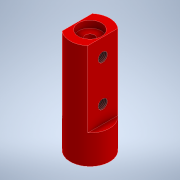
# Autodesk Inventor part: Drum
Saved by Autodesk Inventor 2021 (Build 250183000, 183)
## iProperties
Created: 2022-05-14
Part Number: Drum
Material: Aluminum 6061
Document SubType Name: Modeling
Designer: ermoz
Density: 2.7 g/cm^3
Appearance: Aluminum - Flat
Mass: 135.109 g
Surface Area: 148.591 cm^2
Volume: 50.0405 cm^3
Author: ermoz
Autodesk Inventor part; units mm, degrees
ref_plane "YZ Plane" through (0, 0, 0) normal (1, 0, 0) x (0, 1, 0)
ref_plane "XZ Plane" through (0, 0, 0) normal (0, 1, 0) x (-1, 0, 0)
ref_plane "XY Plane" through (0, 0, 0) normal (0, 0, 1) x (1, 0, 0)
sketch "Sketch1" plane through (0, 0, 0) normal (0, 1, 0) x (-1, 0, 0)
  circle A0 centre (0, 0) radius 4
  circle A1 centre (0, 0) radius 17
  dimension "d0" = 8
  dimension "d1" = 34
  constraints: 2 centre point, 2 coincident
  measures "d0" diameter of A0
  measures "d1" diameter of A1
extrude "Extrusion1" add sketch "Sketch1" along normal blind 90
sketch "Sketch3" plane through (0, 90, 0) normal (0, 1, 0) x (1, 0, 0)
  line L0 (11, 24.9102) -> (-11, 24.9102)
  line L1 (-11, 24.9102) -> (-11, -24.9102)
  line L2 (-11, -24.9102) -> (11, -24.9102)
  line L3 (11, -24.9102) -> (11, 24.9102)
  line L4 (11, 24.9102) -> (-11, -24.9102) construction
  line L5 (-11, 24.9102) -> (11, -24.9102) construction
  circle A0 centre (0, 0) radius 17
  circle A1 centre (0, 0) radius 17 projected
  point P0 (11, 12.9615)
  point P1 (11, -12.9615)
  point P2 (-11, -12.9615)
  point P3 (-11, 12.9615)
  dimension "d7" = 22
  constraints: 12 end point, 2 midpoint, 2 parallel, 1 centre point, 1 coincident, 1 concentric, 1 horizontal, 1 perpendicular
  measures "d7" distance of L1.end L2.end
extrude "Extrusion3" cut sketch "Sketch3" against normal blind 65 contours A0 L3 | L1 A0
sketch "Sketch4" plane through (-11, 90, -12.9615) normal (-1, 0, 0) x (0, 0, 1)
  circle A0 centre (12.9615, -50) radius 4
  circle A1 centre (12.9615, -15) radius 4
  line L0 (0, 0) -> (25.923, 0) projected
  line L1 (29.9615, -90) -> (-4.0385, -90) projected
  line L2 (0, -65) -> (25.923, -65) projected
  line L3 (25.923, 0) -> (25.923, -65) projected
  line L4 (0, 0) -> (25.923, 0) projected
  line L5 (0, -65) -> (0, 0) projected
  line L6 (0, -65) -> (25.923, -65) projected
  line L7 (25.923, 0) -> (25.923, -65) projected
  line L8 (12.9615, -65) -> (12.9615, -59.6994)
  point P0 (0.995, 0)
  point P1 (15.5881, 0)
  dimension "d12" = 15
  dimension "d15" = 8
  dimension "d17" = 15
  constraints: 2 centre point, 2 end point, 1 equal radius, 1 midpoint, 1 point on line, 1 vertical, 1 vertical alignment
  measures "d12" distance from line of L0 A1.centre
  measures "d15" diameter of A0
  measures "d17" distance from line of L2 A0.centre
extrude "Extrusion4" cut sketch "Sketch4" against normal through all contours A0 | A1
sketch "Sketch5" plane through (0, 0, 0) normal (0, -1, 0) x (1, 0, 0)
  circle A0 centre (0, 0) radius 14.5
  dimension "d18" = 29
  constraints: 1 centre point, 1 coincident
  measures "d18" diameter of A0
extrude "Extrusion5" cut sketch "Sketch5" against normal blind 18
thread "Thread1" size "M8x1.25" class "6H" standard "ANSI Metric M Profile" full length
thread "Thread2" size "M8x1.25" class "6H" standard "ANSI Metric M Profile" full length
thread "Thread3" size "M8x1.25" class "6H" standard "ANSI Metric M Profile" full length
thread "Thread4" size "M8x1.25" class "6H" standard "ANSI Metric M Profile" full length
sketch "Sketch6" plane through (0, 90, 0) normal (0, 1, 0) x (1, 0, 0)
  circle A0 centre (0, 0) radius 10
  dimension "d29" = 20
  constraints: 1 centre point, 1 coincident
  measures "d29" diameter of A0
extrude "Extrusion6" cut sketch "Sketch6" against normal blind 6
equation "\"d12\" = d11"
equation "\"d11\" = 15"
body "Solid1"
